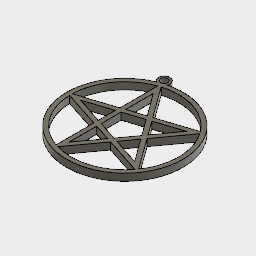
FPROJ_9 (Autodesk Fusion 360 design; units mm, degrees)
Autodesk Fusion 360 part; units mm, degrees
sketch "草图2" plane through (0, 0, 0) normal (0, 1, 0) x (1, 0, 0)
  line L0 (-9.5492, 29.3893) -> (-9.5492, -29.3893)
  line L1 (-9.5492, -29.3893) -> (25, 18.1636)
  line L2 (25, 18.1636) -> (-30.9017, 0)
  line L3 (-30.9017, 0) -> (25, -18.1636)
  line L4 (25, -18.1636) -> (-9.5492, 29.3893)
  line L5 (-37.5985, -0.9785) -> (29.8427, -22.8914)
  line L6 (30.993, -21.3083) -> (-10.688, 36.0607)
  line L7 (-10.688, -36.0607) -> (30.993, 21.3083)
  line L8 (29.8427, 22.8914) -> (-37.5985, 0.9785)
  line L9 (-12.5492, 35.456) -> (-12.5492, -35.456)
  circle A0 centre (0, 0) radius 40.6112
  circle A1 centre (0, 0) radius 37.6112
  dimension "d2" = 3
extrude "拉伸1" add sketch "草图2" along normal blind 5 contours L0 L4 L6 L8 L9 A1 | L0 L2 L4 L8 | L0 L2 L8 L9 | L2 L4 L6 L8 | L0 L2 L3 L9 | L2 L3 L5 L8 L9 A1 | L1 L2 L4 L6 | L1 L2 L6 L7 L8 A1 | L0 L1 L3 L5 | L0 L3 L5 L9 | L1 L3 L4 L7 | L1 L4 L6 L7 | L0 L1 L5 L7 L9 A1 | L1 L3 L5 L7 | L3 L4 L5 L6 L7 A1 | A0 makes body 1
sketch "草图3" plane through (0, 5, 0) normal (0, 1, 0) x (-1, 0, 0)
  arc A0 (10.688, 36.0607) -> (-29.8427, 22.8914) centre (0, 0) ccw
  line L0 (10.688, 36.0607) -> (-4.7933, 14.7524)
  line L1 (-4.7933, 14.7524) -> (-29.8427, 22.8914)
  line L2 (9.5492, -29.3893) -> (-1.7933, -13.7777)
  line L3 (-1.7933, -13.7777) -> (9.5492, -10.0923)
  line L4 (9.5492, -10.0923) -> (9.5492, -29.3893)
  arc A1 (12.5492, -35.456) -> (37.5985, -0.9785) centre (0, 0) ccw
  line L5 (12.5492, -35.456) -> (12.5492, -9.1175)
  line L6 (12.5492, -9.1175) -> (37.5985, -0.9785)
  line L7 (9.5492, 29.3893) -> (9.5492, 10.0923)
  line L8 (9.5492, 10.0923) -> (-1.7933, 13.7777)
  line L9 (-1.7933, 13.7777) -> (9.5492, 29.3893)
  line L10 (-25, 18.1636) -> (-6.6475, 12.2005)
  line L11 (-6.6475, 12.2005) -> (-13.6575, 2.552)
  line L12 (-13.6575, 2.552) -> (-25, 18.1636)
  line L13 (30.9017, 0) -> (12.5492, -5.9631)
  line L14 (12.5492, -5.9631) -> (12.5492, 5.9631)
  line L15 (12.5492, 5.9631) -> (30.9017, 0)
  arc A2 (37.5985, 0.9785) -> (12.5492, 35.456) centre (0, 0) ccw
  line L16 (37.5985, 0.9785) -> (12.5492, 9.1175)
  line L17 (12.5492, 9.1175) -> (12.5492, 35.456)
  line L18 (-25, -18.1636) -> (-13.6575, -2.552)
  line L19 (-13.6575, -2.552) -> (-6.6475, -12.2005)
  line L20 (-6.6475, -12.2005) -> (-25, -18.1636)
  line L21 (-30.993, 21.3083) -> (-15.5116, 0)
  line L22 (-15.5116, 0) -> (-30.993, -21.3083)
  arc A3 (-30.993, 21.3083) -> (-30.993, -21.3083) centre (0, 0) ccw
  arc A4 (-29.8427, -22.8914) -> (10.688, -36.0607) centre (0, 0) ccw
  line L23 (-29.8427, -22.8914) -> (-4.7933, -14.7524)
  line L24 (-4.7933, -14.7524) -> (10.688, -36.0607)
  line L25 (-11.8034, 0) -> (-3.6475, 11.2257)
  line L26 (-3.6475, 11.2257) -> (9.5492, 6.9379)
  line L27 (9.5492, 6.9379) -> (9.5492, -6.9379)
  line L28 (9.5492, -6.9379) -> (-3.6475, -11.2257)
  line L29 (-3.6475, -11.2257) -> (-11.8034, 0)
  circle A5 centre (0, 0) radius 40.6112
  circle A6 centre (-70, 30) radius 2.5
  circle A7 centre (-70, 30) radius 4
extrude "拉伸2" add sketch "草图3" along normal blind 5 separate body contours A7 makes body 2
move_body "移动1" bodies 2 to x (1, 0, 0) y (0, 1, 0) z (0, 0, 1) at (-85, 0, -75)
move_body "移动2" bodies 2 to x (1, 0, 0) y (0, 1, 0) z (0, 0, 1) at (0, -5, 0)
move_body "移动3" bodies 2 to x (1, 0, 0) y (0, 1, 0) z (0, 0, 1) at (1.5742, 0, 3.989)
combine "合并1" operation add target body 1 tool bodies 2
